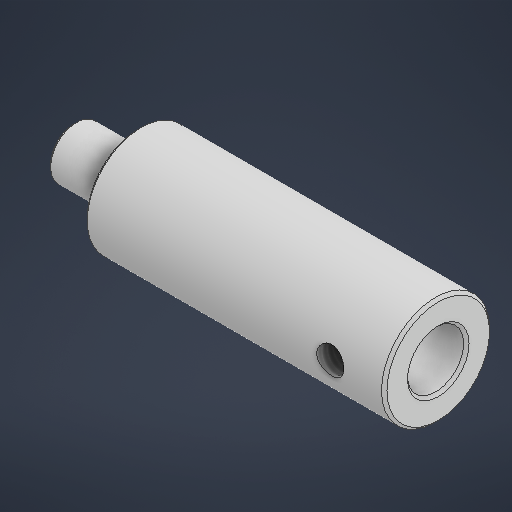
# Autodesk Inventor part: ParrallelShaft
Saved by Autodesk Inventor 2026.3 (Build 303398000, 398)
## iProperties
Created: 2026-05-02
Part Number: ParrallelShaft
Material: Generic
Document SubType Name: Modeling
Designer: frede
Density: 1 g/cm^3
Appearance: Default
Author: frede
Autodesk Inventor part; units mm, degrees
ref_plane "YZ Plane" through (0, 0, 0) normal (1, 0, 0) x (0, 1, 0)
ref_plane "XZ Plane" through (0, 0, 0) normal (0, 1, 0) x (-1, 0, 0)
sketch "Sketch2" plane through (0, 0, 0) normal (0, 1, 0) x (-1, 0, 0)
  line L0 (0.25, 5) -> (27.5, 5)
  line L1 (27.75, 4.75) -> (27.75, 2.4)
  line L2 (27.75, 2.4) -> (33.5, 2.4)
  line L3 (33.75, 2.15) -> (33.75, 0)
  line L4 (9.75, 2.6) -> (0.25, 2.6)
  line L5 (0, 2.85) -> (0, 4.75)
  line L6 (10, 2.35) -> (10, 0)
  line L7 (33.75, 2.15) -> (33.5, 2.4)
  line L8 (27.75, 4.75) -> (27.5, 5)
  line L9 (0.25, 5) -> (0, 4.75)
  line L10 (0, 2.85) -> (0.25, 2.6)
  line L11 (9.75, 2.6) -> (10, 2.35)
  line L12 (33.75, 0) -> (10, 0)
  point P0 (0, 0)
  point P1 (0, 5)
  point P2 (27.75, 5)
  point P3 (33.75, 2.4)
  point P4 (10, 2.6)
  point P5 (0, 2.6)
  dimension "d1" = 27.75
  dimension "d2" = 2.6
  dimension "d3" = 6
  dimension "d4" = 5
  dimension "d5" = 0.25
  dimension "d6" = 0.25
  dimension "d7" = 0.25
  dimension "d8" = 0.25
  dimension "d9" = 0.25
  dimension "d10" = 0.25
  dimension "d11" = 0.25
  dimension "d12" = 0.25
  dimension "d13" = 0.25
  dimension "d14" = 0.25
  constraints: 26 end point, 10 point on line, 3 horizontal, 3 perpendicular, 2 vertical
  measures "d1" distance of point (0, 5) point (27.75, 5)
  measures "d2" distance of point (27.75, 5) L1.end
  measures "d3" distance of L1.end point (33.75, 2.4)
  measures "d4" distance from line of point (0, 0) L0
  measures "d5" distance of L3.start point (33.75, 2.4)
  measures "d6" distance of L2.end point (33.75, 2.4)
  measures "d7" distance of L1.start point (27.75, 5)
  measures "d8" distance of L0.end point (27.75, 5)
  measures "d9" distance of L0.start point (0, 5)
  measures "d10" distance of L5.end point (0, 5)
  measures "d11" distance of L5.start point (0, 2.6)
  measures "d12" distance of L4.end point (0, 2.6)
  measures "d13" distance of L4.start point (10, 2.6)
  measures "d14" distance of L6.start point (10, 2.6)
revolve "Revolution1" add sketch "Sketch2" angle 360 about axis through (-33.75, 0, 0) along (1, 0, 0)
ref_plane "Work Plane1" through (0, 0, 5) normal (0, 0, 1) x (1, 0, 0)
sketch "Sketch3" plane through (0, 0, 5) normal (0, 0, 1) x (1, 0, 0)
  circle A0 centre (-5, 0) radius 1.25
  point P0 (0, 0)
  dimension "d17" = 2.5
  constraints: 1 centre point
  measures "d17" diameter of A0
extrude "Extrusion1" cut sketch "Sketch3" against normal blind 5
thread "Thread1" size "M3x0.5" class "6H" standard "ISO Metric profile" full length
equation "\"d6\" = d5"
equation "\"d7\" = d5"
equation "\"d8\" = d7"
equation "\"d9\" = d5"
equation "\"d10\" = d9"
equation "\"d11\" = d5"
equation "\"d12\" = d11"
equation "\"d14\" = d13"
body "Solid1"
